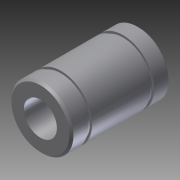
# Autodesk Inventor part: lm8uu
Saved by Autodesk Inventor 2012 (Build 160160000, 160)
## iProperties
Created: 2013-02-05
Part Number: lm8uu
Material: Default
Document SubType Name: Modeling
Designer: mce
Density: 1 g/cm^3
Mass: 2.97771 g
Surface Area: 20.4363 cm^2
Volume: 2.97771 cm^3
Author: mce
Autodesk Inventor part; units mm, degrees
ref_plane "YZ Plane" through (0, 0, 0) normal (1, 0, 0) x (0, 1, 0)
ref_plane "XZ Plane" through (0, 0, 0) normal (0, 1, 0) x (-1, 0, 0)
ref_plane "XY Plane" through (0, 0, 0) normal (0, 0, 1) x (1, 0, 0)
sketch "Sketch1" plane through (0, 0, 0) normal (0, 0, 1) x (1, 0, 0)
  line L0 (0, 21.9424) -> (0, -17.6259)
  line L1 (4, 26.2687) -> (4, 2.2687)
  line L2 (4, 2.2687) -> (7, 2.2687)
  line L3 (7, 2.2687) -> (7.5, 2.7687)
  line L4 (7.5, 2.7687) -> (7.5, 6.2687)
  line L5 (7.5, 6.2687) -> (7, 6.2687)
  line L6 (7, 6.2687) -> (7, 7.2687)
  line L7 (7, 7.2687) -> (7.5, 7.2687)
  line L8 (7.5, 7.2687) -> (7.5, 21.2687)
  line L9 (7.5, 21.2687) -> (7, 21.2687)
  line L10 (7, 21.2687) -> (7, 22.2687)
  line L11 (7, 22.2687) -> (7.5, 22.2687)
  line L12 (7.5, 22.2687) -> (7.5, 25.7687)
  line L13 (7.5, 25.7687) -> (7, 26.2687)
  line L14 (7, 26.2687) -> (4, 26.2687)
  dimension "d1" = 1
  dimension "d2" = 1
  dimension "d3" = 0.5
  dimension "d4" = 0.5
  dimension "d5" = 0.5
  dimension "d6" = 0.5
  dimension "d7" = 24
  dimension "d8" = 8
  dimension "d9" = 15
  dimension "d10" = 4
  dimension "d11" = 4
  dimension "d12" = 0.5
  constraints: 30 end point, 7 horizontal, 7 vertical, 3 collinear
  measures "d1" distance between parallel lines of L11 L9
  measures "d2" distance between parallel lines of L7 L5
  measures "d3" distance from line of L2 L3.end
  measures "d4" distance from line of L4 L2.end
  measures "d5" distance from line of L14 L12.end
  measures "d6" distance from line of L12 L13.end
  measures "d7" distance between parallel lines of L14 L2
  measures "d8" diameter of L1 L0
  measures "d9" diameter of L4 L0
  measures "d10" distance between parallel lines of L5 L2
  measures "d11" distance between parallel lines of L11 L14
  measures "d12" distance between parallel lines of L10 L8
revolve "Revolution1" add sketch "Sketch1" angle 360 about axis through (0, 21.9424, 0) along (0, -1, 0)
body "Solid1"
